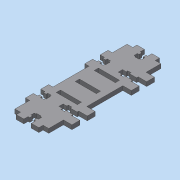
# Autodesk Inventor part: X-Anchor_Bearing_Ring_Top_Single
Saved by Autodesk Inventor 2016 SP1 (Build 200210100, 210)
## iProperties
Created: 2016-01-20
Part Number: X-Anchor_Bearing_Ring_Top_Single
Material: Generic
Document SubType Name: Modeling
Designer: Mohamed A.
Density: 1 g/cm^3
Appearance: Default
Author: Mohamed A.
Autodesk Inventor part; units mm, degrees
ref_plane "YZ Plane" through (0, 0, 0) normal (1, 0, 0) x (0, 1, 0)
ref_plane "XZ Plane" through (0, 0, 0) normal (0, 1, 0) x (-1, 0, 0)
ref_plane "XY Plane" through (0, 0, 0) normal (0, 0, 1) x (1, 0, 0)
sketch "Sketch1" plane through (0, 0, 0) normal (0, 0, 1) x (1, 0, 0)
  line L0 (16.5005, -29.3335) -> (10.5005, -29.3335)
  line L1 (10.5005, -29.3335) -> (10.5005, -39.8335)
  line L2 (16.5005, -23.7335) -> (10.5005, -23.7335)
  line L3 (10.5005, -23.7335) -> (10.5005, -22.5835)
  line L4 (10.5005, -18.4335) -> (16.5005, -18.4335)
  line L5 (16.5005, -23.7335) -> (16.5005, -29.3335)
  line L6 (25.9291, -21.0835) -> (-23.8941, -21.0835) construction
  line L7 (10.5005, -19.5835) -> (5.5005, -19.5835)
  line L8 (0.5005, -19.5835) -> (0.5005, -22.5835)
  line L9 (0.5005, -22.5835) -> (3.1005, -22.5835)
  line L10 (3.1005, -18.4335) -> (5.5005, -18.4335)
  line L11 (5.5005, -18.4335) -> (5.5005, -19.5835)
  line L12 (5.5005, -23.7335) -> (3.1005, -23.7335)
  line L13 (3.1005, -23.7335) -> (3.1005, -22.5835)
  line L14 (10.5005, -19.5835) -> (10.5005, -18.4335)
  line L15 (16.5005, -12.8335) -> (10.5005, -12.8335)
  line L16 (10.5005, -12.8335) -> (10.5005, -6.0102)
  line L17 (16.5005, -12.8335) -> (16.5005, -18.4335)
  line L18 (-29.2331, 0) -> (54.6642, 0) construction
  line L19 (5.5005, -22.5835) -> (5.5005, -23.7335)
  line L20 (3.1005, -19.5835) -> (3.1005, -18.4335)
  line L21 (3.1005, -19.5835) -> (0.5005, -19.5835)
  line L22 (5.5005, -22.5835) -> (10.5005, -22.5835)
  line L23 (16.5005, 29.3335) -> (10.5005, 29.3335)
  line L24 (10.5005, 29.3335) -> (10.5005, 39.8335)
  line L25 (16.5005, 23.7335) -> (10.5005, 23.7335)
  line L26 (10.5005, 23.7335) -> (10.5005, 22.5835)
  line L27 (10.5005, 18.4335) -> (16.5005, 18.4335)
  line L28 (16.5005, 23.7335) -> (16.5005, 29.3335)
  line L29 (10.5005, 19.5835) -> (5.5005, 19.5835)
  line L30 (0.5005, 19.5835) -> (0.5005, 22.5835)
  line L31 (0.5005, 22.5835) -> (3.1005, 22.5835)
  line L32 (3.1005, 18.4335) -> (5.5005, 18.4335)
  line L33 (5.5005, 18.4335) -> (5.5005, 19.5835)
  line L34 (5.5005, 23.7335) -> (3.1005, 23.7335)
  line L35 (3.1005, 23.7335) -> (3.1005, 22.5835)
  line L36 (10.5005, 19.5835) -> (10.5005, 18.4335)
  line L37 (16.5005, 12.8335) -> (10.5005, 12.8335)
  line L38 (10.5005, 12.8335) -> (10.5005, 6.0102)
  line L39 (16.5005, 12.8335) -> (16.5005, 18.4335)
  line L40 (5.5005, 22.5835) -> (5.5005, 23.7335)
  line L41 (3.1005, 19.5835) -> (3.1005, 18.4335)
  line L42 (3.1005, 19.5835) -> (0.5005, 19.5835)
  line L43 (5.5005, 22.5835) -> (10.5005, 22.5835)
  line L44 (10.5005, 6.0102) -> (10.5005, -6.0102)
  line L45 (-16.5005, -29.3335) -> (-13.5005, -29.3335)
  line L46 (-13.5005, -29.3335) -> (-13.5005, -39.8335)
  line L47 (-16.5005, -23.7335) -> (-13.5005, -23.7335)
  line L48 (-13.5005, -23.7335) -> (-13.5005, -22.5835)
  line L49 (-13.5005, -22.5835) -> (-11.5005, -22.5835)
  line L50 (-11.5005, -22.5835) -> (-11.5005, -23.7335)
  line L51 (-11.5005, -23.7335) -> (-9.1005, -23.7335)
  line L52 (-9.1005, -23.7335) -> (-9.1005, -22.5835)
  line L53 (-9.1005, -22.5835) -> (-8.5005, -22.5835)
  line L54 (-8.5005, -22.5835) -> (-8.5005, -19.5835)
  line L55 (-8.5005, -19.5835) -> (-9.1005, -19.5835)
  line L56 (-9.1005, -19.5835) -> (-9.1005, -18.4335)
  line L57 (-9.1005, -18.4335) -> (-11.5005, -18.4335)
  line L58 (-11.5005, -18.4335) -> (-11.5005, -19.5835)
  line L59 (-13.5005, -19.5835) -> (-13.5005, -18.4335)
  line L60 (-16.5005, -18.4335) -> (-13.5005, -18.4335)
  line L61 (-13.5005, -19.5835) -> (-11.5005, -19.5835)
  line L62 (-16.5005, -29.3335) -> (-16.5005, -23.7335)
  line L63 (-16.5005, -12.8335) -> (-13.5005, -12.8335)
  line L64 (-16.5005, -18.4335) -> (-16.5005, -12.8335)
  line L65 (-16.5005, 29.3335) -> (-13.5005, 29.3335)
  line L66 (-13.5005, 29.3335) -> (-13.5005, 39.8335)
  line L67 (-16.5005, 23.7335) -> (-13.5005, 23.7335)
  line L68 (-13.5005, 23.7335) -> (-13.5005, 22.5835)
  line L69 (-13.5005, 22.5835) -> (-11.5005, 22.5835)
  line L70 (-11.5005, 22.5835) -> (-11.5005, 23.7335)
  line L71 (-11.5005, 23.7335) -> (-9.1005, 23.7335)
  line L72 (-9.1005, 23.7335) -> (-9.1005, 22.5835)
  line L73 (-9.1005, 22.5835) -> (-8.5005, 22.5835)
  line L74 (-8.5005, 22.5835) -> (-8.5005, 19.5835)
  line L75 (-8.5005, 19.5835) -> (-9.1005, 19.5835)
  line L76 (-9.1005, 19.5835) -> (-9.1005, 18.4335)
  line L77 (-9.1005, 18.4335) -> (-11.5005, 18.4335)
  line L78 (-11.5005, 18.4335) -> (-11.5005, 19.5835)
  line L79 (-13.5005, 19.5835) -> (-13.5005, 18.4335)
  line L80 (-16.5005, 18.4335) -> (-13.5005, 18.4335)
  line L81 (-13.5005, 19.5835) -> (-11.5005, 19.5835)
  line L82 (-16.5005, 29.3335) -> (-16.5005, 23.7335)
  line L83 (-16.5005, 12.8335) -> (-13.5005, 12.8335)
  line L84 (-16.5005, 18.4335) -> (-16.5005, 12.8335)
  line L85 (-13.5005, 12.8335) -> (-13.5005, -12.8335)
  line L86 (10.5005, -39.8335) -> (6.5003, -39.8335)
  line L87 (6.5003, -39.8335) -> (6.5003, -42.8335)
  line L88 (1.15, -42.8335) -> (1.15, -39.8335)
  line L89 (1.15, -39.8335) -> (0, -39.8335)
  line L90 (0, -39.8335) -> (0, -37.8335)
  line L91 (0, -37.8335) -> (1.15, -37.8335)
  line L92 (1.15, -37.8335) -> (1.15, -35.4335)
  line L93 (1.15, -35.4335) -> (0, -35.4335)
  line L94 (0, -35.4335) -> (0, -34.8335)
  line L95 (0, -34.8335) -> (-3, -34.8335)
  line L96 (-3, -34.8335) -> (-3, -35.4335)
  line L97 (-3, -35.4335) -> (-4.15, -35.4335)
  line L98 (-4.15, -35.4335) -> (-4.15, -37.8335)
  line L99 (-4.15, -37.8335) -> (-3, -37.8335)
  line L100 (-3, -37.8335) -> (-3, -39.8335)
  line L101 (-3, -39.8335) -> (-4.15, -39.8335)
  line L102 (-4.15, -39.8335) -> (-4.15, -42.8335)
  line L103 (-13.5005, -39.8335) -> (-9.5003, -39.8335)
  line L104 (-9.5003, -39.8335) -> (-9.5003, -42.8335)
  line L105 (-1.5, -32.9153) -> (-1.5, -45.3833) construction
  line L106 (6.5003, -42.8335) -> (1.15, -42.8335)
  line L107 (-4.15, -42.8335) -> (-9.5003, -42.8335)
  line L108 (10.5005, 39.8335) -> (6.5003, 39.8335)
  line L109 (6.5003, 39.8335) -> (6.5003, 42.8335)
  line L110 (1.15, 42.8335) -> (1.15, 39.8335)
  line L111 (1.15, 39.8335) -> (0, 39.8335)
  line L112 (0, 39.8335) -> (0, 37.8335)
  line L113 (0, 37.8335) -> (1.15, 37.8335)
  line L114 (1.15, 37.8335) -> (1.15, 35.4335)
  line L115 (1.15, 35.4335) -> (0, 35.4335)
  line L116 (0, 35.4335) -> (0, 34.8335)
  line L117 (0, 34.8335) -> (-3, 34.8335)
  line L118 (-3, 34.8335) -> (-3, 35.4335)
  line L119 (-3, 35.4335) -> (-4.15, 35.4335)
  line L120 (-4.15, 35.4335) -> (-4.15, 37.8335)
  line L121 (-4.15, 37.8335) -> (-3, 37.8335)
  line L122 (-3, 37.8335) -> (-3, 39.8335)
  line L123 (-3, 39.8335) -> (-4.15, 39.8335)
  line L124 (-4.15, 39.8335) -> (-4.15, 42.8335)
  line L125 (-13.5005, 39.8335) -> (-9.5003, 39.8335)
  line L126 (-9.5003, 39.8335) -> (-9.5003, 42.8335)
  line L127 (6.5003, 42.8335) -> (1.15, 42.8335)
  line L128 (-4.15, 42.8335) -> (-9.5003, 42.8335)
  line L129 (5.999, 14.9998) -> (5.999, 11.9998)
  line L130 (5.999, 11.9998) -> (-9.001, 11.9998)
  line L131 (-9.001, 11.9998) -> (-9.001, 14.9998)
  line L132 (-9.001, 14.9998) -> (5.999, 14.9998)
  line L133 (-9.001, -1.5002) -> (-9.001, 1.4998)
  line L134 (-9.001, 1.4998) -> (5.999, 1.4998)
  line L135 (5.999, 1.4998) -> (5.999, -1.5002)
  line L136 (5.999, -1.5002) -> (-9.001, -1.5002)
  line L137 (5.999, -12.0002) -> (5.999, -15.0002)
  line L138 (5.999, -15.0002) -> (-9.001, -15.0002)
  line L139 (-9.001, -15.0002) -> (-9.001, -12.0002)
  line L140 (-9.001, -12.0002) -> (5.999, -12.0002)
  point P0 (0, 0)
  point P1 (-13.5005, 42.8335)
  point P2 (10.5005, 42.8335)
  point P3 (10.5005, -42.8335)
  point P4 (-13.5005, -42.8335)
  dimension "d2" = 6
  dimension "d4" = 5.6
  dimension "d5" = 5.3
  dimension "d6" = 3
  dimension "d8" = 2.4
  dimension "d11" = 16
  dimension "d14" = 3
  dimension "d15" = 5
  dimension "d16" = 8
  dimension "d17" = 24.001
  dimension "d18" = 16.0007
  constraints: 282 end point, 65 symmetric about line, 49 point on line, 37 perpendicular, 22 horizontal, 21 collinear, 14 parallel, 11 equal length, 11 vertical, 17 other
  measures "d2" distance of L0.start L0.end
  measures "d4" distance between parallel lines of L0 L2
  measures "d5" distance between parallel lines of L2 L4
  measures "d6" distance between parallel lines of L9 L7
  measures "d8" distance of L12.start L12.end
  measures "d11" distance between parallel lines of L5 L8
  measures "d14" distance of L45.start L45.end
  measures "d15" distance between parallel lines of L62 L50
  measures "d16" distance between parallel lines of L62 L54
  measures "d17" distance of point (-13.5, -42.833) point (10.501, -42.833)
  measures "d18" distance between parallel lines of L104 L87
extrude "Extrusion1" add sketch "Sketch1" along normal blind 3
equation "\"d18\" = 0.666667 * d17"
body "Solid1"
